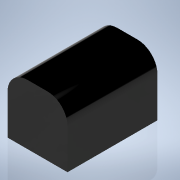
# Autodesk Inventor part: Servo
Saved by Autodesk Inventor 2021 (Build 250183000, 183)
## iProperties
Created: 2021-03-23
Part Number: Servo
Material: Generic
Document SubType Name: Modeling
Designer: calst
Density: 1 g/cm^3
Appearance: Glossy - Black
Author: calst
Autodesk Inventor part; units mm, degrees
ref_plane "YZ Plane" through (0, 0, 0) normal (1, 0, 0) x (0, 1, 0)
ref_plane "XZ Plane" through (0, 0, 0) normal (0, 1, 0) x (-1, 0, 0)
ref_plane "XY Plane" through (0, 0, 0) normal (0, 0, 1) x (1, 0, 0)
sketch "Sketch1" plane through (0, 0, 0) normal (0, 1, 0) x (-1, 0, 0)
  line L0 (-30, 45) -> (30, 45)
  line L1 (30, 45) -> (30, -45)
  line L2 (30, -45) -> (-30, -45)
  line L3 (-30, -45) -> (-30, 45)
  line L4 (-30, 45) -> (30, -45) construction
  line L5 (30, 45) -> (-30, -45) construction
  point P0 (0, 0)
  dimension "d0" = 90
  dimension "d1" = 60
  constraints: 12 end point, 2 midpoint, 2 parallel, 1 horizontal, 1 perpendicular
  measures "d0" distance of L0.end L1.end
  measures "d1" distance of L0.start L0.end
extrude "Extrusion1" add sketch "Sketch1" along normal blind 60
fillet "Fillet1" radius 20 2 edges at (30, 60, 0) (-30, 60, 0)
sketch "Sketch2" plane through (30, 0, -45) normal (0, 0, -1) x (-1, 0, 0)
  circle A0 centre (30, 30) radius 10
  point P0 (30, 0)
  dimension "d6" = 20
  constraints: 1 centre point
  measures "d6" diameter of A0
extrude "Extrusion2" add sketch "Sketch2" along normal blind 15
sketch "Sketch3" plane through (0, 30, -60) normal (0, 0, -1) x (-1, 0, 0)
  circle A0 centre (0, 0) radius 10 projected
  circle A1 centre (0, 10) radius 1
  circle A2 centre (-4.0674, 9.1355) radius 1
  circle A3 centre (-7.4314, 6.6913) radius 1
  circle A4 centre (-9.5106, 3.0902) radius 1
  circle A5 centre (-9.9452, -1.0453) radius 1
  circle A6 centre (-8.6603, -5) radius 1
  circle A7 centre (-5.8779, -8.0902) radius 1
  circle A8 centre (-2.0791, -9.7815) radius 1
  circle A9 centre (2.0791, -9.7815) radius 1
  circle A10 centre (5.8779, -8.0902) radius 1
  circle A11 centre (8.6603, -5) radius 1
  circle A12 centre (9.9452, -1.0453) radius 1
  circle A13 centre (9.5106, 3.0902) radius 1
  circle A14 centre (7.4314, 6.6913) radius 1
  circle A15 centre (4.0674, 9.1355) radius 1
  point P0 (0, -30)
  dimension "d9" = 2
  dimension "d12" = 360
  constraints: 15 centre point, 2 coincident, 1 vertical alignment, 45 other
  measures "d9" diameter of A1
extrude "Extrusion3" cut sketch "Sketch3" against normal blind 30 contours A13 A0 | A0 A13 | A12 A0 | A0 A12 | A14 A0 | A0 A14 | A11 A0 | A0 A11 | A15 A0 | A0 A15 | A10 A0 | A0 A10 | A1 A0 | A0 A1 | A9 A0 | A0 A9 | A2 A0 | A0 A2 | A8 A0 | A0 A8 | A3 A0 | A0 A3 | A7 A0 | A0 A7 | A4 A0 | A0 A4 | A6 A0 | A0 A6 | A5 A0 | A0 A5
sketch "Sketch4" plane through (30, 0, -45) normal (0, 0, -1) x (-1, 0, 0)
  circle A0 centre (30, 30) radius 10.4769
  circle A1 centre (30, 30) radius 10
  line L0 (0, 0) -> (60, 0) projected
  point P0 (30, 0)
  dimension "d16" = 20
  dimension "d19" = 30
  dimension "d20" = 30
  constraints: 2 centre point, 1 coincident
  measures "d16" diameter of A1
  measures "d19" distance of point (30, 0) A1.centre
  measures "d20" distance from line of L0 A0.centre
extrude "Extrusion4" cut sketch "Sketch4" against normal blind 15
body "Solid1"
